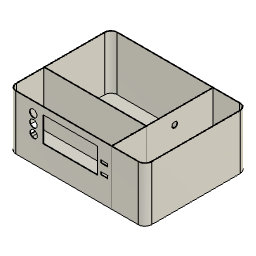
enclosure1 (Autodesk Fusion 360 design; units mm, degrees)
Autodesk Fusion 360 part; units mm, degrees
sketch "Sketch1" plane through (0, 0, 0) normal (0, 0, 1) x (1, 0, 0) in component "Component"
  line L0 (0, 0) -> (50, 0)
  line L1 (50, 0) -> (50, 150)
  line L2 (50, 150) -> (0, 150)
  line L3 (0, 150) -> (0, 0)
  dimension "d1" = 150
  constraint horizontal L0
  constraint vertical L1
  constraint horizontal L2
  constraint vertical L3
  constraint coincident L0.start L3.end
  measures "d1" distance of L0.start L2.end
extrude "Extrude1" add sketch "Sketch1" along normal blind 80 in component "Component"
fillet "Fillet1" radius 10 1 edges at (50, 0, 40) in component "Component"
fillet "Fillet2" radius 10 1 edges at (50, 150, 40) in component "Component"
shell "Shell1" thickness 1 removed faces 1 at (16.6667, 53.3333, 80) in component "Component"
sketch "Sketch2" plane through (1, 0, 0) normal (1, 0, 0) x (0, 1, 0) in component "Component"
  line L0 (1, 1) -> (149, 1)
  line L1 (149, 1) -> (149, 80)
  line L2 (149, 80) -> (1, 80)
  line L3 (1, 80) -> (1, 1)
move_face "OffsetFaces1" offset 150 1 faces at (0, 100, 26.6667) in component "Component"
fillet "Fillet3" radius 10 1 edges at (-150, 0, 40) in component "Component"
fillet "Fillet4" radius 10 1 edges at (-150, 150, 40) in component "Component"
shell "Shell2" thickness 1 removed faces 1 at (-93, 50.3333, 80) in component "Component"
sketch "Sketch3" plane through (0, 0, 1) normal (0, 0, 1) x (-1, 0, 0) in component "Component"
  line L0 (0, -1) -> (0, -149)
  line L1 (0, -149) -> (140, -149)
  arc A0 (140, -149) -> (149, -140) centre (140, -140) ccw
  line L2 (149, -140) -> (149, -10)
  arc A1 (149, -10) -> (140, -1) centre (140, -10) ccw
  line L3 (140, -1) -> (0, -1)
  line L4 (149, -50.0233) -> (-1, -50.0233)
  line L5 (-1, -50.0233) -> (-1, -51.0233)
  line L6 (-1, -51.0233) -> (149, -51.0233)
  line L7 (149, -51.0233) -> (149, -50.0233)
  dimension "d41" = 150
  dimension "d42" = 1
  constraint horizontal L4
  constraint vertical L5
  constraint horizontal L6
  constraint vertical L7
  constraint coincident L2 L4.start
  measures "d41" distance of L4.start L4.end
  measures "d42" distance of L4.start L6.end
extrude "Extrude2" add sketch "Sketch3" along normal blind 80 contours L0 L2 L4 L6 L7 in component "Component"
sketch "Sketch4" plane through (0, 0, 0) normal (0, -1, 0) x (1, 0, 0) in component "Component"
  line L0 (-140, 80) -> (-140, 0)
  line L1 (-140, 0) -> (40, 0)
  line L2 (40, 0) -> (40, 80)
  line L3 (40, 80) -> (-140, 80)
  line L4 (-100, 70) -> (-20, 70)
  line L5 (-20, 70) -> (-20, 33)
  line L6 (-20, 33) -> (-100, 33)
  line L7 (-100, 33) -> (-100, 70)
  line L8 (-15, 70) -> (-5, 70)
  line L9 (-5, 70) -> (-5, 66)
  line L10 (-5, 66) -> (-15, 66)
  line L11 (-15, 66) -> (-15, 70)
  line L12 (-15, 55) -> (-5, 55)
  line L13 (-5, 55) -> (-5, 51)
  line L14 (-5, 51) -> (-15, 51)
  line L15 (-15, 51) -> (-15, 55)
  line L16 (-15, 40) -> (-5, 40)
  line L17 (-5, 40) -> (-5, 36)
  line L18 (-5, 36) -> (-15, 36)
  line L19 (-15, 36) -> (-15, 40)
  dimension "d45" = 37
  dimension "d71" = 10
  constraint horizontal L4
  constraint vertical L5
  constraint horizontal L6
  constraint vertical L7
  constraint horizontal L8
  constraint vertical L9
  constraint horizontal L10
  constraint vertical L11
  constraint horizontal L12
  constraint vertical L13
  constraint horizontal L14
  constraint vertical L15
  constraint horizontal L16
  constraint vertical L17
  constraint horizontal L18
  constraint vertical L19
  measures "d45" distance of L4.start L6.end
  measures "d71" distance of L12.start L12.end
extrude "Extrude7" cut sketch "Sketch4" against normal blind 1 contours L16 L17 L18 L19 in component "Component"
extrude "Extrude6" cut sketch "Sketch4" against normal blind 1 contours L12 L13 L14 L15 in component "Component"
extrude "Extrude3" cut sketch "Sketch4" against normal blind 1 contours L4 L5 L6 L7 in component "Component"
hole "Hole1" at (-114.3363, 0, 64.245) direction (0, 1, 0) diameter 11 depth 1 tip angle 118 in component "Component"
hole "Hole2" at (-113.7358, 0, 38.3229) direction (0, 1, 0) diameter 11 depth 1 tip angle 118 in component "Component"
hole "Hole3" at (-114.1717, 0, 51.3825) direction (0, 1, 0) diameter 11 depth 1 tip angle 118 in component "Component"
hole "Hole4" at (1, 92.7342, 61.0906) direction (-1, 0, 0) diameter 8.3 depth 1 tip angle 118 in component "Component"
hole "Hole5" at (1, 7.4051, 64.4732) direction (-1, 0, 0) diameter 3 depth 1 tip angle 118 in component "Component"
sketch "Sketch5" plane through (0, 50.0233, 0) normal (0, -1, 0) x (1, 0, 0) in component "Component"
  line L0 (-149, 1) -> (0, 1)
  line L1 (0, 1) -> (0, 80)
  line L2 (0, 80) -> (0, 81)
  line L3 (0, 81) -> (-149, 81)
  line L4 (-149, 81) -> (-149, 80)
  line L5 (-149, 80) -> (-149, 1)
  line L6 (-10, 60) -> (-21, 60)
  line L7 (-21, 60) -> (-21, 56)
  line L8 (-21, 56) -> (-10, 56)
  line L9 (-10, 56) -> (-10, 60)
  dimension "d63" = 11
  dimension "d64" = 4
  constraint horizontal L6
  constraint vertical L7
  constraint horizontal L8
  constraint vertical L9
  measures "d63" distance of L6.start L6.end
  measures "d64" distance of L6.start L8.end
extrude "Extrude4" cut sketch "Sketch5" against normal blind 1 contours L6 L7 L8 L9 in component "Component"
sketch "Sketch6" plane through (-150, 0, 0) normal (-1, 0, 0) x (0, -1, 0) in component "Component"
  line L0 (-140, 80) -> (-140, 0)
  line L1 (-140, 0) -> (-10, 0)
  line L2 (-10, 0) -> (-10, 80)
  line L3 (-10, 80) -> (-140, 80)
  line L4 (-45, 5) -> (-30, 5)
  line L5 (-30, 5) -> (-30, 18)
  line L6 (-30, 18) -> (-45, 18)
  line L7 (-45, 18) -> (-45, 5)
  dimension "d67" = 15
  dimension "d68" = 13
  constraint horizontal L4
  constraint vertical L5
  constraint horizontal L6
  constraint vertical L7
  measures "d67" distance of L4.start L4.end
  measures "d68" distance of L4.start L6.end
extrude "Extrude5" cut sketch "Sketch6" against normal blind 1 contours L4 L5 L6 L7 in component "Component"
component "Component" placed x (1, 0, 0) y (0, 1, 0) z (0, 0, 1) at (0, 0, 0)
